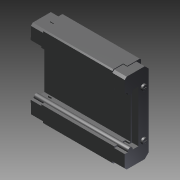
# Autodesk Inventor part: SEBS 9WA Slide
Saved by Autodesk Inventor 2015 SP1 (Build 190203100, 203)
## iProperties
Category: PARTsolutions
Company: NIPPON_BR
Created: 2015-08-08
Part Number: SEBS 9WA Slide
Catalog Web Link: www.cadenas.de
Description: wide blocks, SEBS-WA/WAY 1-
Vendor: NIPPON_BR
Document SubType Name: Modeling
Designer: PARTuser1
Manufacturer: NIPPON_BR
Mass: 6.27549 g
Surface Area: 35.0707 cm^2
Volume: 6.27549 cm^3
Density: 1 g/cm^3
Material: Generic
Appearance: PSOLRGB-192-192-192
PSOL_IDENT_0: {$CADENAS_DATA\23d-libs\nippon_br\slide_guide\seb_a\sebs-wa_way\sebs-wa_way.prj},196 {VTYP=3D},{NB=S
PSOL_IDENT_1: EBS 9WA Slide},{LINA=SEBS 9WA Slide},{NN=wide blocks, SEBS-WA/WAY 1},{DATE=24.03.2015 14:35:04},{GEO
PSOL_IDENT_2: MDATE=24.03.2015 14:32:00},{VERSION=},{LINEID=60},{LINESUBID=-1},{WBVAR=TOP,SS}  {NB=SEBS 9WA Slide}
PSOL_IDENT_3: ,{LINA=SEBS 9WA Slide},{KT=DUMMY},{TOP=},{SS=},{PN=SEBS 9WA},{H=12.000},{W=6.000},{B=30.000},{L1=35.
PSOL_IDENT_4: 900},{L2=38.000},{P1=21.000},{P2=12.000},{S1=M2.6},{LL=3.000},{L3=28.400},{P3=0.000},{S2=0},{S3=M3},
PSOL_IDENT_5: {LL2=0.000},{BB=9.000},{H1=7.500},{C=18.000},{TOP1='','Standard'},{CF=0.400},{CF1=1.410},{NDM=2.600}
PSOL_IDENT_6: ,{KDM=1.567},{UD=5.000},{UD1=1.140},{UD2=2.860},{UD3=1.150},{UD4=11.000},{UD5=12.000},{UD6=17.000},{
PSOL_IDENT_7: UD7=2.450},{UD8=0.500},{UD9=0.200},{UD10=29.500},{UD11=8.500},{UD12=3.750},{UD13=5.250},{UD14=2.000}
PSOL_IDENT_8: ,{UD15=5.700},{ND2='9WAS'},{NDM2=4.000},{KDM2=2.013},{R1=3.000},{R2=0.160},{VD1R=17.000},{VDU=21.820
PSOL_IDENT_9: },{VDV=2.500},{VDE=0.600},{SV=0.000},{SSI=0.000},{SUDR=4.550},{SR=0.800},{SE=0.500},{SEW=0.100},{P=4
PSOL_IDENT_10: .000},{UD16=16.000},{UD17=15.000},{SE1=17.800},{SE2=6.950},{SE3=0.400},{SE4=27.000},{R=0.900},{ER=0.
PSOL_IDENT_11: 900},{ER1=9.250},{ER2=5.000},{UDT=3.000},{NN=3.050},{NN1=1.500},{ND=6.000},{UD122=28.4},{UD133=5.25}
PSOL_IDENT_12: ,{LX=17.95}
NN: 3.050
NB: SEBS 9WA Slide
NBSYN: $PN.$TOP.$SS. Slide
LINA: SEBS 9WA Slide
TOP: Standard
SS: No seal
PN: SEBS 9WA
H: 12.000
W: 6.000
B: 30.000
L1: 35.900
L2: 38.000
P1: 21.000
P2: 12.000
S1: M2.6
LL: 3.000
L3: 28.400
P3: 0.000
S2: 0
S3: M3
LL2: 0.000
BB: 9.000
H1: 7.500
C: 18.000
CF: 0.400
CF1: 1.410
NDM: 2.600
KDM: 1.567
UD: 5.000
UD1: 1.140
UD2: 2.860
UD3: 1.150
UD4: 11.000
UD5: 12.000
UD6: 17.000
UD7: 2.450
UD8: 0.500
UD9: 0.200
UD10: 29.500
UD11: 8.500
UD12: 3.750
UD13: 5.250
UD14: 2.000
UD15: 5.700
ND2: '9WAS'
NDM2: 4.000
KDM2: 2.013
R1: 3.000
R2: 0.160
VD1R: 17.000
VDU: 21.820
VDV: 2.500
VDE: 0.600
SV: 0.000
SSI: 0.000
SUDR: 4.550
SR: 0.800
SE: 0.500
SEW: 0.100
P: 4.000
UD16: 16.000
UD17: 15.000
SE1: 17.800
SE2: 6.950
SE3: 0.400
SE4: 27.000
R: 0.900
ER: 0.900
ER1: 9.250
ER2: 5.000
UDT: 3.000
NN1: 1.500
ND: 6.000
SUPPLIER: NIPPON_BR
ARTICLENO: SEBS 9WA Slide
BOMINFO: SEBS 9WA Slide
CREATOR: CADENAS GmbH
Title: SEBS 9WA Slide
Author: Cadenas PARTsolutions
Autodesk Inventor part; units mm, degrees
sketch "Sketch_29" plane through (-17.95, 0, 0) normal (1, 0, 0) x (0, 0, -1)
  line L0 (-15, 11.6) -> (-15, 3.4)
  line L1 (-15, 3.4) -> (-14.6, 3)
  line L2 (-14.6, 3) -> (14.6, 3)
  line L3 (14.6, 3) -> (15, 3.4)
  line L4 (15, 3.4) -> (15, 11.6)
  line L5 (15, 11.6) -> (14.6, 12)
  line L6 (14.6, 12) -> (-14.6, 12)
  line L7 (-14.6, 12) -> (-15, 11.6)
  constraints: 16 end point
extrude "Extrusion1" add sketch "Sketch_29" along normal blind 35.9
sketch "Sketch2" plane through (-17.95, 12, 14.6) normal (0, 1, 0) x (1, 0, 0)
  point P0 (11.95, 4.1)
hole "Hole1" at (-6, 12, 10.5) direction (0, -1, 0) diameter 2.1129 depth 3.6 tip angle 120 countersink diameter 2.6 countersink angle 90 thread size "M2.6x0.45" class "6H" standard "ISO Metric profile"
sketch "Sketch3" plane through (-17.95, 12, 14.6) normal (0, 1, 0) x (1, 0, 0)
  point P0 (23.95, 4.1)
hole "Hole2" at (6, 12, 10.5) direction (0, -1, 0) diameter 2.1129 depth 3.6 tip angle 120 countersink diameter 2.6 countersink angle 90 thread size "M2.6x0.45" class "6H" standard "ISO Metric profile"
sketch "Sketch4" plane through (-17.95, 12, 14.6) normal (0, 1, 0) x (1, 0, 0)
  point P0 (11.95, 25.1)
hole "Hole3" at (-6, 12, -10.5) direction (0, -1, 0) diameter 2.1129 depth 3.6 tip angle 120 countersink diameter 2.6 countersink angle 90 thread size "M2.6x0.45" class "6H" standard "ISO Metric profile"
sketch "Sketch5" plane through (-17.95, 12, 14.6) normal (0, 1, 0) x (1, 0, 0)
  point P0 (23.95, 25.1)
hole "Hole4" at (6, 12, -10.5) direction (0, -1, 0) diameter 2.1129 depth 3.6 tip angle 120 countersink diameter 2.6 countersink angle 90 thread size "M2.6x0.45" class "6H" standard "ISO Metric profile"
sketch "Sketch_23" plane through (14.2, 0, 0) normal (1, 0, 0) x (0, 0, -1)
  line L0 (-15, 2.25) -> (15, 2.25)
  line L1 (15, 2.25) -> (15, 12)
  line L2 (15, 12) -> (-15, 12)
  line L3 (-15, 12) -> (-15, 2.25)
  line L4 (-14.75, 10.34) -> (-14.75, 3.705)
  line L5 (-14.75, 3.705) -> (-14.045, 3)
  line L6 (-14.045, 3) -> (14.045, 3)
  line L7 (14.045, 3) -> (14.75, 3.705)
  line L8 (14.75, 3.705) -> (14.75, 10.34)
  line L9 (14.75, 10.34) -> (13.34, 11.75)
  line L10 (13.34, 11.75) -> (-13.34, 11.75)
  line L11 (-13.34, 11.75) -> (-14.75, 10.34)
  constraints: 24 end point
extrude "Extrusion2" cut sketch "Sketch_23" along normal blind 28.4
sketch "Sketch_26" plane through (-14.2, 0, 0) normal (1, 0, 0) x (0, 0, -1)
  line L0 (-15, 2.25) -> (15, 2.25)
  line L1 (15, 2.25) -> (15, 12)
  line L2 (15, 12) -> (-15, 12)
  line L3 (-15, 12) -> (-15, 2.25)
  line L4 (-14.75, 10.34) -> (-14.75, 3.705)
  line L5 (-14.75, 3.705) -> (-14.045, 3)
  line L6 (-14.045, 3) -> (14.045, 3)
  line L7 (14.045, 3) -> (14.75, 3.705)
  line L8 (14.75, 3.705) -> (14.75, 10.34)
  line L9 (14.75, 10.34) -> (13.34, 11.75)
  line L10 (13.34, 11.75) -> (-13.34, 11.75)
  line L11 (-13.34, 11.75) -> (-14.75, 10.34)
  constraints: 24 end point
extrude "Extrusion3" cut sketch "Sketch_26" against normal blind 28.4
sketch "Sketch_39" plane through (-17.95, 0, 0) normal (1, 0, 0) x (0, 0, -1)
  line L0 (-15, 7) -> (-15, 2)
  line L1 (-15, 2) -> (15, 2)
  line L2 (15, 2) -> (15, 7)
  line L3 (15, 7) -> (14.75, 7)
  line L4 (14.75, 7) -> (14.75, 3.705)
  line L5 (14.75, 3.705) -> (14.045, 3)
  line L6 (14.045, 3) -> (-14.045, 3)
  line L7 (-14.045, 3) -> (-14.75, 3.705)
  line L8 (-14.75, 3.705) -> (-14.75, 7)
  line L9 (-14.75, 7) -> (-15, 7)
  constraints: 20 end point
extrude "Extrusion4" cut sketch "Sketch_39" along normal blind 5.25
sketch "Sketch_40" plane through (17.95, 0, 0) normal (1, 0, 0) x (0, 0, -1)
  line L0 (-15, 7) -> (-15, 2)
  line L1 (-15, 2) -> (15, 2)
  line L2 (15, 2) -> (15, 7)
  line L3 (15, 7) -> (14.75, 7)
  line L4 (14.75, 7) -> (14.75, 3.705)
  line L5 (14.75, 3.705) -> (14.045, 3)
  line L6 (14.045, 3) -> (-14.045, 3)
  line L7 (-14.045, 3) -> (-14.75, 3.705)
  line L8 (-14.75, 3.705) -> (-14.75, 7)
  line L9 (-14.75, 7) -> (-15, 7)
  constraints: 20 end point
extrude "Extrusion5" cut sketch "Sketch_40" against normal blind 5.25
sketch "Sketch_42" plane through (-17.95, 0, 0) normal (1, 0, 0) x (0, 0, -1)
  line L0 (-6, 12) -> (-5.5, 11.75)
  line L1 (-5.5, 11.75) -> (5.5, 11.75)
  line L2 (5.5, 11.75) -> (6, 12)
  line L3 (6, 12) -> (-6, 12)
  constraints: 8 end point
extrude "Extrusion6" cut sketch "Sketch_42" along normal blind 38
sketch "Sketch_107" plane through (-17.95, 0, 0) normal (1, 0, 0) x (0, 0, -1)
  line L0 (-15, 3) -> (15, 3)
  line L1 (15, 3) -> (15, 12)
  line L2 (15, 12) -> (-15, 12)
  line L3 (-15, 12) -> (-15, 3)
  circle A0 centre (8.5, 9.8) radius 1
  circle A1 centre (-8.5, 9.8) radius 1
  constraints: 8 end point, 2 centre point
extrude "Extrusion7" cut sketch "Sketch_107" along normal blind 0.7
sketch "Sketch_108" plane through (17.95, 0, 0) normal (1, 0, 0) x (0, 0, -1)
  line L0 (-15, 3) -> (15, 3)
  line L1 (15, 3) -> (15, 12)
  line L2 (15, 12) -> (-15, 12)
  line L3 (-15, 12) -> (-15, 3)
  circle A0 centre (8.5, 9.8) radius 1
  circle A1 centre (-8.5, 9.8) radius 1
  constraints: 8 end point, 2 centre point
extrude "Extrusion8" cut sketch "Sketch_108" against normal blind 0.7
sketch "Sketch_109" plane through (-17.95, 0, 0) normal (1, 0, 0) x (0, 0, -1)
  line L0 (-9.1, 9.7) -> (-8.6, 9.7)
  line L1 (-8.6, 9.7) -> (-8.6, 9.2)
  line L2 (-8.6, 9.2) -> (-8.4, 9.2)
  line L3 (-8.4, 9.2) -> (-8.4, 9.7)
  line L4 (-8.4, 9.7) -> (-7.9, 9.7)
  line L5 (-7.9, 9.7) -> (-7.9, 9.9)
  line L6 (-7.9, 9.9) -> (-8.4, 9.9)
  line L7 (-8.4, 9.9) -> (-8.4, 10.4)
  line L8 (-8.4, 10.4) -> (-8.6, 10.4)
  line L9 (-8.6, 10.4) -> (-8.6, 9.9)
  line L10 (-8.6, 9.9) -> (-9.1, 9.9)
  line L11 (-9.1, 9.9) -> (-9.1, 9.7)
  constraints: 24 end point
extrude "Extrusion9" cut sketch "Sketch_109" along normal blind 0.4
sketch "Sketch_110" plane through (-17.95, 0, 0) normal (1, 0, 0) x (0, 0, -1)
  line L0 (7.9, 9.9) -> (7.9, 9.7)
  line L1 (7.9, 9.7) -> (8.4, 9.7)
  line L2 (8.4, 9.7) -> (8.4, 9.2)
  line L3 (8.4, 9.2) -> (8.6, 9.2)
  line L4 (8.6, 9.2) -> (8.6, 9.7)
  line L5 (8.6, 9.7) -> (9.1, 9.7)
  line L6 (9.1, 9.7) -> (9.1, 9.9)
  line L7 (9.1, 9.9) -> (8.6, 9.9)
  line L8 (8.6, 9.9) -> (8.6, 10.4)
  line L9 (8.6, 10.4) -> (8.4, 10.4)
  line L10 (8.4, 10.4) -> (8.4, 9.9)
  line L11 (8.4, 9.9) -> (7.9, 9.9)
  constraints: 24 end point
extrude "Extrusion10" cut sketch "Sketch_110" along normal blind 0.4
sketch "Sketch_111" plane through (17.95, 0, 0) normal (1, 0, 0) x (0, 0, -1)
  line L0 (-9.1, 9.7) -> (-8.6, 9.7)
  line L1 (-8.6, 9.7) -> (-8.6, 9.2)
  line L2 (-8.6, 9.2) -> (-8.4, 9.2)
  line L3 (-8.4, 9.2) -> (-8.4, 9.7)
  line L4 (-8.4, 9.7) -> (-7.9, 9.7)
  line L5 (-7.9, 9.7) -> (-7.9, 9.9)
  line L6 (-7.9, 9.9) -> (-8.4, 9.9)
  line L7 (-8.4, 9.9) -> (-8.4, 10.4)
  line L8 (-8.4, 10.4) -> (-8.6, 10.4)
  line L9 (-8.6, 10.4) -> (-8.6, 9.9)
  line L10 (-8.6, 9.9) -> (-9.1, 9.9)
  line L11 (-9.1, 9.9) -> (-9.1, 9.7)
  constraints: 24 end point
extrude "Extrusion11" cut sketch "Sketch_111" against normal blind 0.4
sketch "Sketch_112" plane through (17.95, 0, 0) normal (1, 0, 0) x (0, 0, -1)
  line L0 (7.9, 9.9) -> (7.9, 9.7)
  line L1 (7.9, 9.7) -> (8.4, 9.7)
  line L2 (8.4, 9.7) -> (8.4, 9.2)
  line L3 (8.4, 9.2) -> (8.6, 9.2)
  line L4 (8.6, 9.2) -> (8.6, 9.7)
  line L5 (8.6, 9.7) -> (9.1, 9.7)
  line L6 (9.1, 9.7) -> (9.1, 9.9)
  line L7 (9.1, 9.9) -> (8.6, 9.9)
  line L8 (8.6, 9.9) -> (8.6, 10.4)
  line L9 (8.6, 10.4) -> (8.4, 10.4)
  line L10 (8.4, 10.4) -> (8.4, 9.9)
  line L11 (8.4, 9.9) -> (7.9, 9.9)
  constraints: 24 end point
extrude "Extrusion12" cut sketch "Sketch_112" against normal blind 0.4
sketch "Sketch_113" plane through (0, 0, 8.5) normal (0, 0, 1) x (1, 0, 0)
  line L0 (-17.85, 9.8) -> (-18.05, 9.8)
  line L1 (-18.05, 10.7) -> (-17.85, 10.8)
  line L2 (-17.85, 10.8) -> (-18.05, 10.8)
  line L3 (-18.05, 10.8) -> (-18.05, 10.7)
  constraints: 8 end point
revolve "Revolution1" cut sketch "Sketch_113" angle 360 about axis through (-17.85, 9.8, 8.5) along (1, 0, 0)
sketch "Sketch_114" plane through (0, 0, -8.5) normal (0, 0, 1) x (1, 0, 0)
  line L0 (-17.85, 9.8) -> (-18.05, 9.8)
  line L1 (-18.05, 10.7) -> (-17.85, 10.8)
  line L2 (-17.85, 10.8) -> (-18.05, 10.8)
  line L3 (-18.05, 10.8) -> (-18.05, 10.7)
  constraints: 8 end point
revolve "Revolution2" cut sketch "Sketch_114" angle 360 about axis through (-17.85, 9.8, -8.5) along (1, 0, 0)
sketch "Sketch_115" plane through (0, 0, 8.5) normal (0, 0, 1) x (1, 0, 0)
  line L0 (18.05, 9.8) -> (17.85, 9.8)
  line L1 (17.85, 10.8) -> (18.05, 10.7)
  line L2 (18.05, 10.7) -> (18.05, 10.8)
  line L3 (18.05, 10.8) -> (17.85, 10.8)
  constraints: 8 end point
revolve "Revolution3" cut sketch "Sketch_115" angle 360 about axis through (18.05, 9.8, 8.5) along (1, 0, 0)
sketch "Sketch_116" plane through (0, 0, -8.5) normal (0, 0, 1) x (1, 0, 0)
  line L0 (18.05, 9.8) -> (17.85, 9.8)
  line L1 (17.85, 10.8) -> (18.05, 10.7)
  line L2 (18.05, 10.7) -> (18.05, 10.8)
  line L3 (18.05, 10.8) -> (17.85, 10.8)
  constraints: 8 end point
revolve "Revolution4" cut sketch "Sketch_116" angle 360 about axis through (18.05, 9.8, -8.5) along (1, 0, 0)
sketch "Sketch_121" plane through (-17.95, 0, 0) normal (1, 0, 0) x (0, 0, -1)
  line L0 (-15, 3) -> (-10.4, 3)
  line L1 (-10.4, 3) -> (-10.4, 8.7)
  line L2 (-10.4, 8.7) -> (10.4, 8.7)
  line L3 (10.4, 8.7) -> (10.4, 3)
  line L4 (10.4, 3) -> (15, 3)
  line L5 (15, 3) -> (15, 12)
  line L6 (15, 12) -> (-15, 12)
  line L7 (-15, 12) -> (-15, 3)
  circle A0 centre (8.5, 9.8) radius 1
  circle A1 centre (-8.5, 9.8) radius 1
  constraints: 16 end point, 2 centre point
extrude "Extrusion13" cut sketch "Sketch_121" along normal blind 0.75
sketch "Sketch_20" plane through (-17.95, 0, 0) normal (1, 0, 0) x (0, 0, -1)
  arc A0 (-9.5, 4.1354) -> (-9.5, 5.8646) centre (-9.25, 5) ccw
  line L0 (-9.5, 4.1354) -> (-9.5, 1.41)
  line L1 (-9.5, 1.41) -> (-8.09, 0)
  line L2 (-8.09, 0) -> (8.09, 0)
  line L3 (8.09, 0) -> (9.5, 1.41)
  line L4 (9.5, 1.41) -> (9.5, 4.1354)
  arc A1 (9.5, 5.8646) -> (9.5, 4.1354) centre (9.25, 5) ccw
  line L5 (9.5, 5.8646) -> (9.5, 8)
  line L6 (9.5, 8) -> (-9.5, 8)
  line L7 (-9.5, 8) -> (-9.5, 5.8646)
  constraints: 16 end point, 4 point on circle, 2 centre point
extrude "Extrusion14" cut sketch "Sketch_20" along normal blind 3.05
sketch "Sketch_21" plane through (17.95, 0, 0) normal (1, 0, 0) x (0, 0, -1)
  arc A0 (-9.5, 4.1354) -> (-9.5, 5.8646) centre (-9.25, 5) ccw
  line L0 (-9.5, 4.1354) -> (-9.5, 1.41)
  line L1 (-9.5, 1.41) -> (-8.09, 0)
  line L2 (-8.09, 0) -> (8.09, 0)
  line L3 (8.09, 0) -> (9.5, 1.41)
  line L4 (9.5, 1.41) -> (9.5, 4.1354)
  arc A1 (9.5, 5.8646) -> (9.5, 4.1354) centre (9.25, 5) ccw
  line L5 (9.5, 5.8646) -> (9.5, 8)
  line L6 (9.5, 8) -> (-9.5, 8)
  line L7 (-9.5, 8) -> (-9.5, 5.8646)
  constraints: 16 end point, 4 point on circle, 2 centre point
extrude "Extrusion15" cut sketch "Sketch_21" against normal blind 3.05
sketch "Sketch_24" plane through (-14.9, 0, 0) normal (1, 0, 0) x (0, 0, -1)
  arc A0 (-9.5, 4.1354) -> (-9.5, 5.8646) centre (-9.25, 5) ccw
  line L0 (-9.5, 4.1354) -> (-9.5, 1.41)
  line L1 (-9.5, 1.41) -> (-8.09, 0)
  line L2 (-8.09, 0) -> (8.09, 0)
  line L3 (8.09, 0) -> (9.5, 1.41)
  line L4 (9.5, 1.41) -> (9.5, 4.1354)
  arc A1 (9.5, 5.8646) -> (9.5, 4.1354) centre (9.25, 5) ccw
  line L5 (9.5, 5.8646) -> (9.5, 7)
  line L6 (9.5, 7) -> (-9.5, 7)
  line L7 (-9.5, 7) -> (-9.5, 5.8646)
  constraints: 16 end point, 4 point on circle, 2 centre point
extrude "Extrusion16" cut sketch "Sketch_24" along normal blind 1.5
sketch "Sketch_22" plane through (-17.95, 0, 0) normal (1, 0, 0) x (0, 0, -1)
  arc A0 (-9, 4.1354) -> (-9, 5.8646) centre (-9.25, 5) ccw
  line L0 (-9, 4.1354) -> (-9, 1.41)
  line L1 (-9, 1.41) -> (-7.59, 0)
  line L2 (-7.59, 0) -> (7.59, 0)
  line L3 (7.59, 0) -> (9, 1.41)
  line L4 (9, 1.41) -> (9, 4.1354)
  arc A1 (9, 5.8646) -> (9, 4.1354) centre (9.25, 5) ccw
  line L5 (9, 5.8646) -> (9, 7.5)
  line L6 (9, 7.5) -> (-9, 7.5)
  line L7 (-9, 7.5) -> (-9, 5.8646)
  constraints: 16 end point, 4 point on circle, 2 centre point
extrude "Extrusion17" cut sketch "Sketch_22" along normal blind 35.9
sketch "Sketch_25" plane through (14.9, 0, 0) normal (1, 0, 0) x (0, 0, -1)
  arc A0 (-9.5, 4.1354) -> (-9.5, 5.8646) centre (-9.25, 5) ccw
  line L0 (-9.5, 4.1354) -> (-9.5, 1.41)
  line L1 (-9.5, 1.41) -> (-8.09, 0)
  line L2 (-8.09, 0) -> (8.09, 0)
  line L3 (8.09, 0) -> (9.5, 1.41)
  line L4 (9.5, 1.41) -> (9.5, 4.1354)
  arc A1 (9.5, 5.8646) -> (9.5, 4.1354) centre (9.25, 5) ccw
  line L5 (9.5, 5.8646) -> (9.5, 7)
  line L6 (9.5, 7) -> (-9.5, 7)
  line L7 (-9.5, 7) -> (-9.5, 5.8646)
  constraints: 16 end point, 4 point on circle, 2 centre point
extrude "Extrusion18" cut sketch "Sketch_25" against normal blind 1.5
ref_plane "sebs_way_p_XY" through (-17.95, 0, 0) normal (1, 0, 0) x (0, 0, -1)
ref_plane "sebs_way_p_YZ" through (-17.95, 0, 0) normal (0, 0, -1) x (0, 1, 0)
ref_plane "sebs_way_p_ZX" through (-17.95, 0, 0) normal (0, 1, 0) x (1, 0, 0)
body "Solid1"
